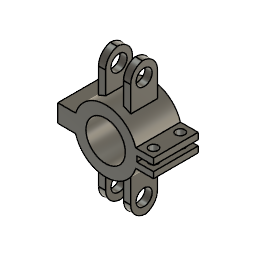
ex1 (Autodesk Fusion 360 design; units mm, degrees)
part number: 2026-04-20-18-09-25-110
Autodesk Fusion 360 part; units mm, degrees
note: some values were not read from the file. Chosen so that the rebuilt part matches the saved one: which pieces of a blend or face edit are solid.
sketch "Piesa" plane through (0, 0, 0) normal (0, 1, 0) x (1, 0, 0)
  circle A0 centre (0, 0) radius 22
  circle A1 centre (0, 0) radius 35
  line L0 (0, 0) -> (50, 0) construction
  line L1 (50, 0) -> (50, -3) construction
  line L2 (50, -3) -> (50, 3) construction
  line L3 (0, 0) -> (0, -60) construction
  line L4 (0, -60) -> (43.5, -60) construction
  line L5 (0, -70) -> (53.5, -70) construction
  line L6 (53.5, 0.1472) -> (53.5, -70) construction
  line L7 (53.5, -10.1603) -> (53.5, 9.8397) construction
  line L8 (33.5429, -9.9939) -> (53.5, -10.1603)
  line L9 (33.5976, 9.8081) -> (53.5, 9.8397)
  line L10 (34.8712, 3) -> (53.5, 3)
  line L11 (34.8712, -3) -> (53.5, -2.9169)
  line L12 (53.5, -10.1603) -> (53.5, -2.9169)
  line L13 (53.5, 3) -> (53.5, 9.8397)
  line L14 (0, -50) -> (-53.5, -50) construction
  line L15 (-53.5, -50) -> (-53.5, 0) construction
  line L16 (-53.5, -10.1984) -> (-53.5, 9.8016) construction
  line L17 (-53.5, -10.1984) -> (-33.4812, -10.1984)
  line L18 (-53.5, 9.8016) -> (-33.5995, 9.8016)
  line L19 (-53.5, -10.1984) -> (-53.5, 9.8016)
  line L20 (-90, 0) -> (-90, -58) construction
  line L21 (-90, 0) -> (-90, -75) construction
  line L22 (0, -70) -> (10, -70) construction
  line L23 (-90, -75) -> (0, -75) construction
  line L24 (0, -75) -> (-10, -75) construction
  line L25 (-10, -33.541) -> (-10, -75)
  line L26 (-10, -75) -> (-18, -75)
  line L27 (-18, -75) -> (-18, -30.0167)
  line L28 (0, -75) -> (10, -75) construction
  line L29 (10, -75) -> (10, -33.541)
  line L30 (10, -75) -> (18, -75)
  line L31 (18, -75) -> (18, -30.0167)
  line L32 (-114.7578, -75) -> (-114.7578, 40) construction
  line L33 (-114.7578, -75) -> (-114.7578, 75) construction
  line L34 (-18, 30.0167) -> (-18, 75)
  line L35 (-114.7578, 75) -> (-18, 75) construction
  line L36 (-18, 75) -> (-10, 75)
  line L37 (-10, 75) -> (-10, 33.541)
  line L38 (-10, 75) -> (60, 75) construction
  line L39 (10, 33.541) -> (10, 75)
  line L40 (10, 75) -> (18, 75)
  line L41 (18, 75) -> (18, 30.0167)
  dimension "d1" = 44
  dimension "d2" = 70
  dimension "d3" = 6
  dimension "d4" = 43.5
  dimension "d5" = 53.5
  dimension "d6" = 20
  dimension "d7" = 53.5
  dimension "d8" = 20
  dimension "d9" = 20.0188
  dimension "d10" = 53.5
  dimension "d11" = 58
  dimension "d12" = 75
  dimension "d13" = 8
  dimension "d14" = 10
  dimension "d15" = 8
  dimension "d17" = 150
  dimension "d18" = 8
  dimension "d19" = 8
  dimension "d20" = 18
  dimension "d21" = 28
  dimension "d22" = 75
  dimension "d23" = 18
  dimension "d24" = 75
  dimension "d25" = 28
  dimension "d26" = 9.7137
  dimension "d27" = 89.522
  dimension "d28" = 0.734
  dimension "d29" = 0.569
  dimension "d30" = 3.1556
  dimension "d31" = 3
  constraint coincident A0.centre A1.centre
  constraint concentric A0 A1
  constraint horizontal L0
  constraint perpendicular L0 L1
  constraint perpendicular L0 L2
  constraint perpendicular L0 L3
  constraint perpendicular L3 L4
  constraint perpendicular L3 L5
  constraint perpendicular L5 L6
  constraint coincident L6 L7.start
  constraint parallel L6 L7
  constraint coincident A1 L8.start
  constraint coincident A1 L9.start
  constraint coincident A1 L10.start
  constraint coincident L7 L10.end
  constraint perpendicular L7 L10
  constraint coincident A1 L11.start
  constraint coincident L7 L11.end
  constraint coincident L3 L14.start
  constraint perpendicular L3 L14
  constraint perpendicular L14 L15
  constraint coincident L15 L16.start
  constraint perpendicular L14 L16
  constraint coincident A1 L17.end
  constraint perpendicular L15 L17
  constraint coincident A1 L18.end
  constraint perpendicular L16 L18
  constraint parallel L15 L20
  constraint parallel L20 L21
  constraint coincident L5 L22.end
  constraint perpendicular L21 L23
  constraint coincident L23 L24.end
  constraint coincident A1 L25.start
  constraint perpendicular L24 L25
  constraint perpendicular L25 L26
  constraint coincident A1 L27.end
  constraint perpendicular L14 L27
  constraint perpendicular L27 L28
  constraint coincident A1 L29.end
  constraint perpendicular L4 L29
  constraint perpendicular L29 L30
  constraint coincident A1 L31.end
  constraint perpendicular L30 L31
  constraint perpendicular L14 L32
  constraint perpendicular L14 L33
  constraint coincident A1 L34.start
  constraint parallel L27 L34
  constraint perpendicular L33 L35
  constraint perpendicular L34 L36
  constraint coincident A1 L37.end
  constraint perpendicular L36 L37
  constraint perpendicular L37 L38
  constraint coincident A1 L39.start
  constraint coincident L38 L39.end
  constraint perpendicular L38 L39
  constraint perpendicular L39 L40
  constraint coincident A1 L41.end
  constraint perpendicular L40 L41
  measures "d1" diameter of A0
  measures "d2" diameter of A1
  measures "d3" distance of L1.end L2.end
  measures "d4" distance of L3.end L4.end
  measures "d5" distance of L5.start L5.end
  measures "d6" distance of L7.start L7.end
  measures "d7" distance of L14.start L14.end
  measures "d8" distance of L16.start L16.end
  measures "d9" distance of L16.start L17.end
  measures "d10" distance of A0.centre L7
  measures "d11" distance of L20.start L20.end
  measures "d12" distance of L20.start L21.end
  measures "d13" distance of L24.end L26.end
  measures "d14" distance of L23.end L28.end
  measures "d15" distance of L28.end L30.end
  measures "d17" distance of L32.start L33.end
  measures "d18" distance of L34.end L36.end
  measures "d19" distance of L39.end L40.end
  measures "d20" distance of A0.centre L34
  measures "d21" distance of L37 L41
  measures "d22" distance of A0.centre L36
  measures "d23" distance of A0.centre L27
  measures "d24" distance of A0.centre L23
  measures "d25" distance of L25 L31
  measures "d26" distance of A0.centre L8
  measures "d27" angle of L8 L31
  measures "d28" angle of L8 L11
  measures "d29" angle of L8 L9
  measures "d30" distance of A0.centre L11
  measures "d31" distance of A0.centre L10
extrude "Extrude4" add sketch "Piesa" along normal blind 25 and the other way blind 25 contours A1 | A1 L9 L10 L13 | A1 L8 L11 L12 | A1 L17 L18 L19
extrude "Extrude5" add sketch "Piesa" along normal blind 15 and the other way blind 15 contours A1 L39 L40 L41 | A1 L29 L30 L31 | A1 L34 L36 L37 | A1 L25 L26 L27
sketch "Filet mic" plane through (0, 0, 0) normal (0, 0, 1) x (1, 0, 0)
  line L0 (53.4004, 24.984) -> (53.4004, 14.984) construction
  line L1 (53.4004, 14.984) -> (43.4004, 14.984)
  circle A0 centre (43.4004, 14.984) radius 5
  line L2 (53.5245, -25.0186) -> (53.5245, -15.0186) construction
  line L3 (53.5245, -15.0186) -> (43.5245, -15.0186) construction
  circle A1 centre (43.5245, -15.0186) radius 5
  dimension "d65" = 10
  dimension "d66" = 10
  dimension "d67" = 10
  dimension "d68" = 10
  dimension "d69" = 10
  dimension "d70" = 10
  constraint vertical L0
  constraint perpendicular L0 L1
  constraint coincident L1.end A0.centre
  constraint vertical L2
  constraint perpendicular L2 L3
  constraint coincident L3.end A1.centre
  measures "d65" distance of L0.start L0.end
  measures "d66" distance of L0.end L1.end
  measures "d67" diameter of A0
  measures "d68" distance of L2.start L2.end
  measures "d69" distance of L2.end L3.end
  measures "d70" diameter of A1
extrude "Extrude6" cut sketch "Filet mic" along normal blind 20 and the other way blind 20
sketch "Folet mare" plane through (0, 0, 0) normal (1, 0, 0) x (0, 1, 0)
  line L0 (0, 0) -> (0, 58) construction
  circle A0 centre (0, 58) radius 9
  line L1 (0, 0) -> (0, -58) construction
  circle A1 centre (0, -58) radius 9
  dimension "d75" = 58
  dimension "d76" = 18
  dimension "d77" = 58
  dimension "d78" = 18
  constraint coincident L0.start L1.start
  constraint vertical L0
  constraint coincident L0.end A0.centre
  constraint parallel L0 L1
  constraint coincident L1.end A1.centre
  measures "d75" distance of L0.start L0.end
  measures "d76" diameter of A0
  measures "d77" distance of L0.start L1.end
  measures "d78" diameter of A1
extrude "Extrude7" cut sketch "Folet mare" along normal blind 30 and the other way blind 30
fillet "Fillet1" radius 17 8 edges at (14, 15, 75) (14, -15, 75) (-14, 15, 75) (-14, -15, 75) (14, -15, -75) (14, 15, -75) (-14, -15, -75) (-14, 15, -75)
named bodies: "Piesa"
